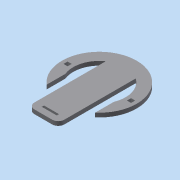
# Autodesk Inventor part: central
Saved by Autodesk Inventor 2015 (Build 190159000, 159)
## iProperties
Created: 2017-10-02
Part Number: central
Material: Generic
Document SubType Name: Modeling
Designer: macbook
Density: 1 g/cm^3
Appearance: Default
Author: macbook
Autodesk Inventor part; units mm, degrees
ref_plane "YZ Plane" through (0, 0, 0) normal (1, 0, 0) x (0, 1, 0)
ref_plane "XZ Plane" through (0, 0, 0) normal (0, 1, 0) x (-1, 0, 0)
ref_plane "XY Plane" through (0, 0, 0) normal (0, 0, 1) x (1, 0, 0)
sketch "Sketch1" plane through (0, 0, 0) normal (0, 0, 1) x (1, 0, 0)
  circle A0 centre (0, 0) radius 50
  circle A1 centre (0, 0) radius 35
  line L0 (-20, 45) -> (20, 45)
  line L1 (20, 45) -> (20, -75)
  line L2 (20, -75) -> (-20, -75)
  line L3 (-20, -75) -> (-20, 45)
  line L4 (-32.4459, -13.125) -> (-32.4459, -38.0429)
  line L5 (32.4459, -13.125) -> (32.4459, -38.0429)
  line L6 (-10, -67) -> (10, -67)
  line L7 (10, -67) -> (10, -64)
  line L8 (10, -64) -> (-10, -64)
  line L9 (-10, -64) -> (-10, -67)
  dimension "d0" = 100
  dimension "d1" = 70
  dimension "d4" = 40
  dimension "d5" = 120
  dimension "d9" = 20
  dimension "d10" = 3
  constraints: 20 end point, 4 parallel, 4 point on circle, 2 centre point, 2 coincident, 2 horizontal, 2 perpendicular, 2 vertical
  measures "d0" diameter of A0
  measures "d1" diameter of A1
  measures "d4" distance of L1.end L2.end
  measures "d5" distance of L0.end L1.end
  measures "d9" distance of L8.end L7.end
  measures "d10" distance of L7.end L6.end
extrude "Extrusion2" add sketch "Sketch1" along normal blind 5.5 contours A0 L5 A1 L1 L0 L3 L4 | L3 A1 L1 A0 | A0 L1 L2 L3 | L3 A1 L1 | L3 L0 L1 A1 | L9 L8 L7 L6
fillet "Fillet1" radius 8 2 edges at (20, -75, 2.75) (-20, -75, 2.75)
sketch "Sketch2" plane through (0, 0, 5.5) normal (0, 0, 1) x (1, 0, 0)
  line L0 (-10, -67) -> (10, -67)
  line L1 (10, -67) -> (10, -64)
  line L2 (10, -64) -> (-10, -64)
  line L3 (-10, -64) -> (-10, -67)
  point P0 (0, 0)
  dimension "d11" = 20
  dimension "d12" = 3
  constraints: 8 end point, 2 parallel, 1 horizontal, 1 perpendicular
  measures "d11" distance of L2.end L1.end
  measures "d12" distance of L1.end L0.end
extrude "Extrusion3" cut sketch "Sketch2" against normal blind 5.5
sketch "Sketch4" plane through (0, 0, 5.5) normal (0, 0, 1) x (1, 0, 0)
  line L0 (39.75, 2.75) -> (45.25, 2.75)
  line L1 (45.25, 2.75) -> (45.25, -2.75)
  line L2 (45.25, -2.75) -> (39.75, -2.75)
  line L3 (39.75, -2.75) -> (39.75, 2.75)
  line L4 (-39.75, -2.75) -> (-45.25, -2.75)
  line L5 (-45.25, -2.75) -> (-45.25, 2.75)
  line L6 (-45.25, 2.75) -> (-39.75, 2.75)
  line L7 (-39.75, 2.75) -> (-39.75, -2.75)
  point P0 (0, 0)
  point P1 (0, 0)
  dimension "d24" = 5.5
  dimension "d25" = 5.5
  dimension "d26" = 360
  constraints: 16 end point, 2 parallel, 1 horizontal, 1 perpendicular, 17 other
  measures "d24" distance of L1.end L2.end
  measures "d25" distance of L0.end L1.end
extrude "Extrusion5" cut sketch "Sketch4" against normal blind 10
body "Solid2"
